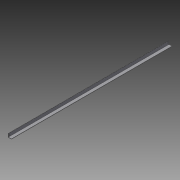
# Autodesk Inventor part: Y_Rail-SquareBar-Rev3
Saved by Autodesk Inventor 2015 (Build 190159000, 159)
## iProperties
Created: 2017-01-10
Part Number: Y_Rail-SquareBar-Rev3
Material: Generic
Document SubType Name: Modeling
Designer: Guy
Density: 1 g/cm^3
Appearance: Default
Mass: 222.064 g
Surface Area: 1563.73 cm^2
Volume: 222.064 cm^3
Author: Guy
Autodesk Inventor part; units mm, degrees
ref_plane "YZ Plane" through (0, 0, 0) normal (1, 0, 0) x (0, 1, 0)
ref_plane "XZ Plane" through (0, 0, 0) normal (0, 1, 0) x (-1, 0, 0)
ref_plane "XY Plane" through (0, 0, 0) normal (0, 0, 1) x (1, 0, 0)
sketch "Sketch1" plane through (0, 0, 0) normal (0, 0, 1) x (1, 0, 0)
  line L0 (0, 0) -> (0, 30)
  line L1 (0, 30) -> (3, 30)
  line L2 (3, 30) -> (3, 3)
  line L3 (3, 3) -> (30, 3)
  line L4 (30, 3) -> (30, 0)
  line L5 (30, 0) -> (0, 0)
  dimension "d0" = 30
  dimension "d1" = 30
  dimension "d2" = 3
  dimension "d3" = 3
  constraints: 12 end point, 5 perpendicular, 1 vertical
  measures "d0" distance between parallel lines of L0 L4
  measures "d1" distance between parallel lines of L5 L1
  measures "d2" distance between parallel lines of L0 L2
  measures "d3" distance between parallel lines of L5 L3
extrude "Extrusion1" add sketch "Sketch1" along normal blind 1450.85
sketch "Sketch3" plane through (3, 3, 0) normal (1, 0, 0) x (0, 0, -1)
  line L0 (0, 27) -> (0, 0) projected
  line L1 (0, 27) -> (-1450.85, 27) projected
  line L2 (-1450.85, 0) -> (-1450.85, 27) projected
  line L3 (0, 0) -> (-1450.85, 0) projected
  circle A0 centre (-10, 17) radius 2.5
  circle A1 centre (-10, 7) radius 2.5
  circle A2 centre (-1440.85, 17) radius 2.5
  circle A3 centre (-1440.85, 7) radius 2.5
  point P0 (0, -3)
  dimension "d20" = 5
  dimension "d21" = 5
  dimension "d22" = 10
  dimension "d23" = 10
  dimension "d24" = 10
  dimension "d25" = 10
  dimension "d28" = 5
  dimension "d29" = 5
  dimension "d30" = 10
  dimension "d31" = 10
  dimension "d32" = 10
  dimension "d33" = 10
  constraints: 4 centre point
  measures "d20" diameter of A1
  measures "d21" diameter of A0
  measures "d22" distance from line of L1 A0.centre
  measures "d23" distance of A1.centre A0.centre
  measures "d24" distance from line of L0 A0.centre
  measures "d25" distance from line of L0 A1.centre
  measures "d28" diameter of A2
  measures "d29" diameter of A3
  measures "d30" distance from line of L2 A2.centre
  measures "d31" distance from line of L2 A3.centre
  measures "d32" distance from line of L1 A2.centre
  measures "d33" distance of A3.centre A2.centre
extrude "Extrusion3" cut sketch "Sketch3" against normal blind 1300 contours A0 | A1 | A2 | A3
body "Solid1"
